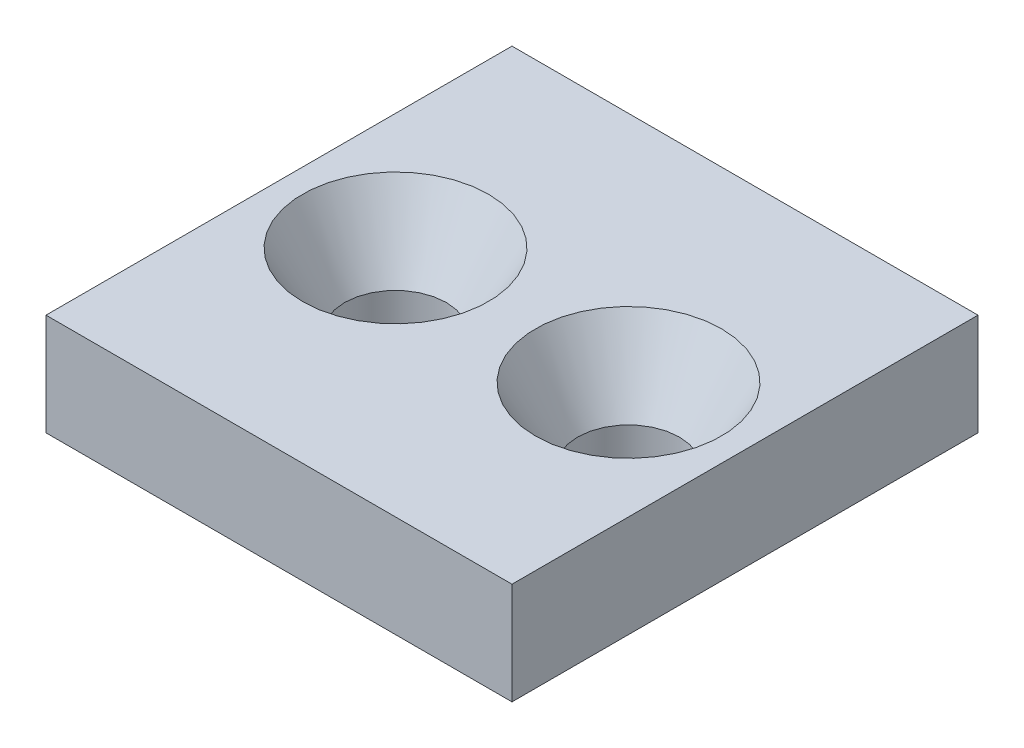
# Autodesk Inventor part: Parte 6_16ME
Saved by Autodesk Inventor 2021 (Build 250183000, 183)
## iProperties
Created: 2020-10-13
Part Number: Parte 6_16ME
Material: Steel, Alloy
Document SubType Name: Modeling
Designer: Erandi
Density: 7.73 g/cm^3
Appearance: Violet
Author: Erandi
Autodesk Inventor part; units mm, degrees
ref_plane "YZ Plane" through (0, 0, 0) normal (1, 0, 0) x (0, 1, 0)
ref_plane "XZ Plane" through (0, 0, 0) normal (0, 1, 0) x (-1, 0, 0)
ref_plane "XY Plane" through (0, 0, 0) normal (0, 0, 1) x (1, 0, 0)
sketch "Sketch1" plane through (0, 0, 0) normal (0, 1, 0) x (-1, 0, 0)
  line L0 (14.0075, -16) -> (-17.9925, -16)
  line L1 (-17.9925, -16) -> (-17.9925, 16)
  line L2 (-17.9925, 16) -> (14.0075, 16)
  line L3 (14.0075, 16) -> (14.0075, -16)
  line L4 (17.4158, 0) -> (-35.0729, 0) construction
  point P0 (0, 0)
  dimension "d0" = 32
  dimension "d1" = 32
  dimension "d2" = 16
  constraints: 10 end point, 2 horizontal, 2 parallel, 1 perpendicular, 1 point on line
  measures "d0" distance of L0.start L0.end
  measures "d1" distance of L0.end L1.end
  measures "d2" distance from line of L4 L0.end
extrude "Extrusion1" add sketch "Sketch1" against normal blind 7
ref_plane "Work Plane1" through (9.9925, 0, 16) normal (1, 0, 0) x (0, 0, -1)
sketch "Sketch2" plane through (9.9925, 0, 16) normal (1, 0, 0) x (0, 0, -1)
  line L0 (16, 0) -> (16, -5)
  line L1 (32, 0) -> (0, 0) projected
  line L2 (19.5, 0) -> (16, 0)
  line L3 (16, -5) -> (19.5, -5)
  line L4 (19.5, 0) -> (16, 0)
  line L5 (19.5, -5) -> (22.3868, 0)
  line L6 (22.3868, 0) -> (16, 0)
  point P0 (19.4027, 0)
  dimension "d9" = 5
  dimension "d17" = 60
  dimension "d18" = 3.5
  constraints: 12 end point, 2 collinear, 2 point on line, 1 horizontal, 1 perpendicular, 1 vertical
  measures "d9" distance of L0.start L0.end
  measures "d17" angle of L5 L1
  measures "d18" distance of L0.end L3.end
revolve "Revolution1" cut sketch "Sketch2" angle 360 about axis through (9.9925, 0, 0) along (0, -1, 0)
pattern_linear "Rectangular Pattern3" count 2 spacing 16 along (-1, 0, 0) of "Revolution1"
sketch "Sketch4" plane through (-6.0075, -5, 0) normal (0, 1, 0) x (1, 0, 0)
  circle A0 centre (0, 0) radius 3.5
  circle A1 centre (16, 0) radius 3.5
  point P0 (6.0075, 0)
  dimension "d31" = 7
  dimension "d32" = 7
  dimension "d35" = 16
  constraints: 2 centre point
  measures "d31" diameter of A0
  measures "d32" diameter of A1
  measures "d35" distance of A1.centre A0.centre
extrude "Extrusion3" cut sketch "Sketch4" against normal blind 2
body "Solid1"
